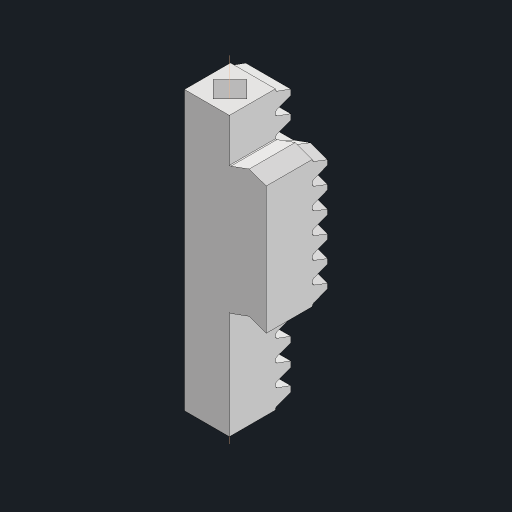
# Autodesk Inventor part: Rack
Saved by Autodesk Inventor 2023.2 (Build 272271030, 271C)
## iProperties
Created: 2023-11-19
Part Number: Rack
Material: Generic
Document SubType Name: Modeling
Designer: robpl
Density: 1 g/cm^3
Appearance: Default
Author: robpl
## iProperties of the stored document Rack_3DPrint.ipt
Created: 2023-11-27
Part Number: Rack_3DPrint
Material: Generic
Document SubType Name: Modeling
Designer: robpl
Density: 1 g/cm^3
Appearance: Default
Author: robpl
Autodesk Inventor part; units mm, degrees
ref_plane "YZ Plane" through (0, 0, 0) normal (1, 0, 0) x (0, 1, 0)
ref_plane "XZ Plane" through (0, 0, 0) normal (0, 1, 0) x (-1, 0, 0)
ref_plane "XY Plane" through (0, 0, 0) normal (0, 0, 1) x (1, 0, 0)
sketch "Sketch1" plane through (0, 0, 0) normal (0, 0, 1) x (1, 0, 0)
  line L0 (0, 0) -> (-12, 0)
  line L1 (-12, 0) -> (-12, 40.840704)
  line L2 (-12, 40.840704) -> (0, 40.840704)
  line L3 (0, 40.840704) -> (0, 0)
  dimension "d0" = 12
  dimension "d1" = 40.8407
  constraints: 8 end point, 2 parallel, 1 horizontal, 1 perpendicular
  measures "d0" distance of L1.end L2.end
  measures "d1" distance of L0.end L1.end
extrude "Extrusion1" add sketch "Sketch1" along normal blind 9
sketch "Sketch2" plane through (-12, 0, 0) normal (1, 0, 0) x (0, 0, -1)
  line L0 (0, 0) -> (0, 40.840704)
  line L1 (0, 40.840704) -> (-9, 40.840704)
  line L2 (-9, 0) -> (-9, 40.840704)
  line L3 (0, 0) -> (-9, 0)
  line L4 (0, 1.149368) -> (-2.25, 0.330435)
  line L5 (-2.25, 0.330435) -> (-2.25, -0.330435)
  line L6 (-2.25, -0.330435) -> (0, -1.149368)
  line L7 (0, -1.149368) -> (0, 1.149368)
  line L8 (-1, -0.785398) -> (-1, 0.785398)
  line L9 (0, 0) -> (-9, 0)
  arc A0 (-2.25, -0.064357) -> (-1.999968, -0.42144) centre (-1.87, -0.064357) ccw
  arc A1 (-1.999968, 0.42144) -> (-2.25, 0.064357) centre (-1.87, 0.064357) ccw
  point P0 (-2.25, 0)
  point P1 (0, 0)
  point P2 (-2.25, 0)
  dimension "d4" = 1
  dimension "d5" = 1.25
  dimension "d6" = 1.5708
  dimension "d7" = 70
  dimension "d17" = 0.38
  constraints: 10 end point, 8 point on line, 4 point on circle, 4 tangent, 3 vertical, 2 centre point, 1 equal length, 1 equal radius, 1 midpoint
  measures "d4" distance between parallel lines of L0 L8
  measures "d5" distance between parallel lines of L5 L8
  measures "d6" distance of L8.start L8.end
  measures "d7" angle of L6 L8
  measures "d17" radius of A0
sketch "Sketch3" plane through (0, 0, 0) normal (0, 0, -1) x (-1, 0, 0)
  line L0 (12, -1.149368) -> (12, 1.149368)
  line L1 (12, -1.149368) -> (5, -1.149368)
  line L2 (5, -1.149368) -> (2.5, -0.239443)
  line L3 (2.5, -0.239443) -> (0, -1.149368)
  point P0 (0, 0)
  dimension "d27" = 7
  dimension "d28" = 5
  dimension "d29" = 20
  constraints: 6 end point, 1 equal length, 1 horizontal, 1 point on line
  measures "d27" distance of L0.start L1.end
  measures "d28" distance of L1.end L3.end
  measures "d29" angle of L1 L2
sweep "Sweep1" cut profiles "Sketch2" path "Sketch3" path curves L1 L2 L3 contours L3 L8 L4 L0 | L7 L6 L8 L3 | L8 L6 A0 L5 L3 | L3 L5 A1 L4 L8
pattern_linear "Rectangular Pattern1" count 14 spacing 3.141593 along (0, 1, 0) of "Sweep1"
sketch "Sketch4" plane through (-12, 40.840704, 9) normal (0, 1, 0) x (1, 0, 0)
  line L0 (10.970457, 7.000032) -> (9.5, 8.38181)
  line L1 (9.5, 8.38181) -> (8.029543, 7.000032)
  line L2 (6.985501, 6.75) -> (0, 6.75)
  line L3 (0, 6.75) -> (0, 0)
  line L4 (12, 0) -> (0, 0)
  line L5 (12, 6.750032) -> (12, 0)
  ellipse E0 centre (12.014499, 7.13) end of major axis (10.903453, 7.13) minor radius 0.38 (10.970457, 7.000032) -> (12, 6.750032) ccw
  ellipse E1 centre (6.985501, 7.13) end of major axis (8.096547, 7.13) minor radius 0.38 (6.985501, 6.75) -> (8.029543, 7.000032) ccw
  line L6 (3.3, 5.849874) -> (0.825126, 3.375)
  line L7 (0.825126, 3.375) -> (3.3, 0.900126)
  line L8 (3.3, 0.900126) -> (5.774874, 3.375)
  line L9 (5.774874, 3.375) -> (3.3, 5.849874)
  line L10 (3.3, 5.849874) -> (3.3, 0.900126) construction
  line L11 (0.825126, 3.375) -> (5.774874, 3.375) construction
  line L12 (0, 6.75) -> (0, 0)
  point P0 (12, 9)
  point P1 (0, 3.375)
  point P2 (3.3, 3.375)
  point P3 (3.3, 3.375)
  point P4 (0, 3.375)
  dimension "d60" = 3.5
  dimension "d61" = 3.3
  constraints: 12 end point, 5 midpoint, 2 parallel, 2 perpendicular, 1 horizontal, 1 horizontal alignment, 2 other
  measures "d60" distance between parallel lines of L6 L8
  measures "d61" distance between parallel lines of L3 L10
sketch "Sketch8" plane through (0, 0, 0) normal (0, 0, -1) x (-1, 0, 0)
  line L0 (0, 40.840704) -> (12, 40.840704)
  line L1 (12, 40.840704) -> (12, 0)
  line L2 (12, 0) -> (0, 0)
  line L3 (0, 0) -> (0, 40.840704)
  line L4 (2.5, 16.623166) -> (0, 15.71324)
  line L5 (5.191317, 15.643607) -> (2.5, 16.623166)
  line L6 (12, 15.643607) -> (5.191317, 15.643607)
  line L7 (2.5, 35.609695) -> (0, 34.69977)
  line L8 (5.214012, 34.621876) -> (2.5, 35.609695)
  line L9 (12, 34.621876) -> (5.214012, 34.621876)
  line L10 (12, 0) -> (0, 0)
  line L11 (5.405329, 0) -> (5.405329, 40.840704)
  point P0 (5.405329, 38.84848)
  point P1 (5.405329, 34.621876)
  point P2 (5.405329, 15.643607)
  constraints: 3 point on line, 2 end point, 1 vertical
extrude "Extrusion7" cut sketch "Sketch8" against normal up to surface (2.25 mm away) contours L0 L11 L9 L8 L7 L3 | L4 L5 L6 L11 L2 L3
extrude "Extrusion8" cut sketch "Sketch4" against normal through all contours L9 L8 L7 L6
sketch "Sketch9" plane through (0, 34.562796, 2.25) normal (0, 0, -1) x (-1, 0, 0)
  line L0 (12, 0.059079) -> (5.405329, 0.059079)
  line L1 (5.405329, 0.059079) -> (5.405329, 3.071959)
  line L2 (12, 3.071959) -> (5.405329, 3.071959)
  line L3 (12, 3.200672) -> (5.405329, 3.200672)
  line L4 (5.405329, 3.200672) -> (5.405329, 6.213552)
  line L5 (12, 6.213552) -> (5.405329, 6.213552)
  line L6 (0, 6.277908) -> (12, 6.277908)
  line L7 (0, 0) -> (0, 6.277908)
  line L8 (2.5, 0.909926) -> (0, 0)
  line L9 (5.191317, -0.069634) -> (2.5, 0.909926)
  line L10 (12, -0.069634) -> (5.191317, -0.069634)
  line L11 (12, -34.49844) -> (5.405329, -34.49844)
  line L12 (5.405329, -34.49844) -> (5.405329, -31.48556)
  line L13 (12, -31.48556) -> (5.405329, -31.48556)
  line L14 (12, -31.356847) -> (5.405329, -31.356847)
  line L15 (5.405329, -31.356847) -> (5.405329, -28.343968)
  line L16 (12, -28.343968) -> (5.405329, -28.343968)
  line L17 (12, -28.215255) -> (5.405329, -28.215255)
  line L18 (5.405329, -28.215255) -> (5.405329, -25.202375)
  line L19 (12, -25.202375) -> (5.405329, -25.202375)
  line L20 (12, -25.073662) -> (5.405329, -25.073662)
  line L21 (5.405329, -25.073662) -> (5.405329, -22.060782)
  line L22 (12, -22.060782) -> (5.405329, -22.060782)
  line L23 (12, -21.932069) -> (5.405329, -21.932069)
  line L24 (5.405329, -21.932069) -> (5.405329, -18.91919)
  line L25 (12, -18.91919) -> (5.405329, -18.91919)
  line L26 (12, -18.790477) -> (5.214012, -18.790477)
  line L27 (5.214012, -18.790477) -> (2.5, -17.802657)
  line L28 (2.5, -17.802657) -> (0, -18.712582)
  line L29 (0, -34.562796) -> (0, -18.712582)
  line L30 (12, -34.562796) -> (0, -34.562796)
  line L31 (0, 6.277908) -> (10.5, 6.277908)
  line L32 (5.405329, 6.277908) -> (5.405329, -34.562796)
  line L33 (10.5, -34.562796) -> (0, -34.562796)
  line L34 (5.405329, -34.49844) -> (5.405329, -31.48556)
  line L35 (12, -34.49844) -> (12, -34.562796)
  line L36 (12, -31.356847) -> (12, -31.48556)
  line L37 (12, -28.215255) -> (12, -28.343968)
  line L38 (12, -25.073662) -> (12, -25.202375)
  line L39 (12, -21.932069) -> (12, -22.060782)
  line L40 (12, -18.790477) -> (12, -18.91919)
  line L41 (12, 0.059079) -> (12, -0.069634)
  line L42 (12, 3.200672) -> (12, 3.071959)
  line L43 (12, 6.277908) -> (12, 6.213552)
  point P0 (5.405329, -18.790477)
  point P1 (5.405329, -0.069634)
  point P2 (5.405329, 6.277908)
  constraints: 2 end point, 2 point on line, 1 collinear
extrude "Extrusion9" cut sketch "Sketch9" against normal through all contours L32 L10 L9 L8 L7 L6 L4 L1 | L32 L30 L29 L28 L27 L26 L24 L21 L18 L15 L12
equation "\"d5\" = 1.25 * d4"
equation "\"d6\" = 1.5708 * d4"
equation "\"d17\" = 0.38 * d4"
body "Solid1"
